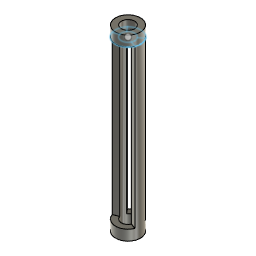
Sleeves (Autodesk Fusion 360 design; units mm, degrees)
Autodesk Fusion 360 part; units mm, degrees
note: some values were not read from the file. Set by a fixed rule: which face or edge a step refers to.
sketch "Sketch1" plane through (0, 0, 0) normal (0, 0, 1) x (1, 0, 0)
  circle A0 centre (0, 0) radius 3.2
  circle A1 centre (0, 0) radius 6
  line L0 (-3.0605, -0.9346) -> (-5.6926, -1.8959)
  line L1 (-2.5603, 1.9196) -> (-4.3765, 4.1044)
  line L2 (2.5603, 1.9196) -> (4.7149, 3.7108)
  line L3 (2.9267, -1.2939) -> (5.5727, -2.2237)
  dimension "d1" = 6.4
  dimension "d2" = 12
  constraint coincident A0 L0.start
  constraint coincident A1 L0.end
  constraint coincident A0 L1.start
  constraint coincident A1 L1.end
  constraint coincident A0 L2.start
  constraint coincident A1 L2.end
  constraint perpendicular L1 L2
  constraint coincident A0 L3.start
  constraint coincident A1 L3.end
  measures "d1" diameter of A0
  measures "d2" diameter of A1
extrude "Extrude1" add sketch "Sketch1" along normal blind 5 contours A0 A1 L2 L3 | A0 A1 L1 L2 | A0 A1 L0 L3 | A0 A1 L0 L1
extrude "Extrude2" add sketch "Sketch1" against normal blind 76 contours A0 A1 L2 L3 | A0 A1 L0 L1
extrude "Extrude3" add sketch "Sketch1" against normal blind 5 from surface at -76 contours A0 A1 L2 L3 | A0 A1 L1 L2 | A0 A1 L0 L3 | A0 A1 L0 L1
